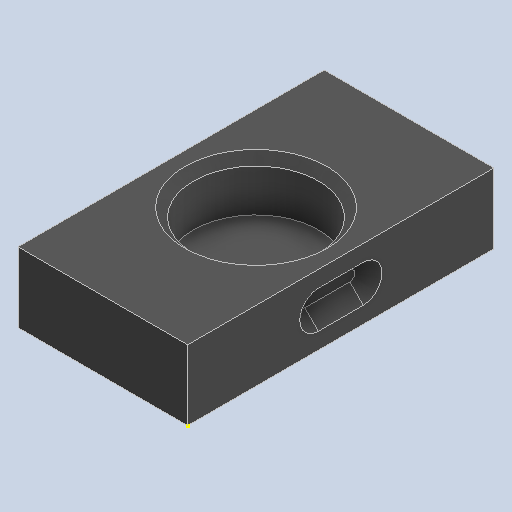
# Autodesk Inventor part: Pieza1
Saved by Autodesk Inventor 2026 (Build 300175050, 175E)
## iProperties
Created: 2025-09-26
Part Number: Pieza1
Material: Plastico PETG
Document SubType Name: Modeling
Designer: bello
Density: 1.27 g/cm^3
Appearance: Genérico
Author: bello
Autodesk Inventor part; units mm, degrees
ref_plane "YZ Plane" through (0, 0, 0) normal (1, 0, 0) x (0, 1, 0)
ref_plane "XZ Plane" through (0, 0, 0) normal (0, 1, 0) x (-1, 0, 0)
sketch "Boceto1" plane through (0, 0, 0) normal (0, 1, 0) x (-1, 0, 0)
  line L0 (0, 0) -> (-50.2, 0)
  line L1 (-50.2, 0) -> (-50.2, -90.6)
  line L2 (-50.2, -90.6) -> (0, -90.6)
  line L3 (0, -90.6) -> (0, 0)
  dimension "d0" = 50.2
  dimension "d1" = 90.6
  constraints: 8 end point, 2 parallel, 1 horizontal, 1 perpendicular
  measures "d0" distance of L2.end L1.end
  measures "d1" distance of L0.end L1.end
extrude "Extrusión1" add sketch "Boceto1" along normal blind 20.7
sketch "Boceto2" plane through (0, 20.7, 0) normal (0, 1, 0) x (1, 0, 0)
  line L0 (-14.4985, 45.3) -> (58.2485, 45.3)
  circle A0 centre (25.1, 45.3) radius 18.5
  line L1 (50.2, 90.6) -> (0, 90.6) projected
  point P0 (0, 0)
  dimension "d7" = 37
  dimension "d51" = 90.6
  dimension "d52" = 0
  constraints: 2 end point, 1 centre point
  measures "d7" diameter of A0
  measures "d51" diameter of L1 L0
  measures "d52" distance from line of A0.centre L0
extrude "Extrusión2" cut sketch "Boceto2" against normal blind 15
sketch "Boceto3" plane through (50.2, 0, 0) normal (1, 0, 0) x (0, 0, -1)
  line L0 (45.3, 28.8672) -> (45.3, -9.3744)
  line L1 (-5.2256, 10.35) -> (70.0589, 10.35)
  line L2 (38.65, 10.35) -> (51.95, 10.35) construction
  line L3 (38.65, 8.85) -> (51.95, 8.85)
  line L4 (51.95, 11.85) -> (38.65, 11.85)
  arc A0 (38.65, 11.85) -> (38.65, 8.85) centre (38.65, 10.35) ccw
  arc A1 (51.95, 8.85) -> (51.95, 11.85) centre (51.95, 10.35) ccw
  line L5 (90.6, 0) -> (90.6, 20.7) projected
  point P0 (0, 0)
  point P1 (45.3, 10.35)
  point P2 (53.45, 10.35)
  point P3 (37.15, 10.35)
  dimension "d11" = 16.3
  dimension "d12" = 3
  dimension "d13" = 0
  dimension "d53" = 45.3
  constraints: 12 end point, 6 point on circle, 4 tangent, 2 centre point, 2 point on line, 1 midpoint, 1 parallel
  measures "d11" distance of point (53.45, 10.35) point (37.15, 10.35)
  measures "d12" distance between parallel lines of L3 L4
  measures "d13" distance from line of point (45.3, 10.35) L0
  measures "d53" distance between parallel lines of L0 L5
extrude "Extrusión3" cut sketch "Boceto3" against normal blind 4
chamfer "Chaflán1" distance 4 angle 45 4 edges at (50.2, 8.85, -45.3) (50.2, 10.35, -37.15) (50.2, 11.85, -45.3) (50.2, 10.35, -53.45)
sketch "Boceto4" plane through (50.2, 0, 0) normal (1, 0, 0) x (0, 0, -1)
  point P0 (0, 0)
ref_plane "Plano de trabajo1" through (25.1, 0, 0) normal (1, 0, 0) x (0, 0, -1)
mirror "Simetría1" about plane through (25.1, 0, 0) normal (1, 0, 0) of "Extrusión3"
chamfer "Chaflán2" distance 4 angle 45 4 edges at (0, 11.85, -45.3) (0, 10.35, -37.15) (0, 8.85, -45.3) (0, 10.35, -53.45)
chamfer "Chaflán3" distance 2.5 angle 45 1 edges at (6.6, 20.7, -45.3)
sketch "Boceto5" plane through (0, 0, 0) normal (0, -1, 0) x (1, 0, 0)
  line L0 (25.1, 22.2035) -> (25.1, -86.3829)
  line L1 (-10.0483, -45.3) -> (59.9656, -45.3)
  circle A0 centre (6.05, -7.2) radius 3.2
  circle A1 centre (44.15, -7.2) radius 3.2
  circle A2 centre (44.15, -83.4) radius 3.2
  line L2 (0, 0) -> (50.2, 0) projected
  circle A3 centre (6.05, -83.4) radius 3.2
  dimension "d35" = 38.1
  dimension "d36" = 38.1
  dimension "d42" = 6.4
  dimension "d46" = 76.2
  dimension "d47" = 76.2
  dimension "d54" = 45.3
  constraints: 4 centre point, 4 end point, 3 equal radius, 2 vertical
  measures "d35" distance of A0.centre A1.centre
  measures "d36" diameter of A0.centre L0
  measures "d42" diameter of A0
  measures "d46" distance of A2.centre A1.centre
  measures "d47" diameter of A1.centre L1
  measures "d54" distance between parallel lines of L1 L2
extrude "Extrusión4" add sketch "Boceto5" along normal blind 4.2
fillet "Empalme1" radius 3.2 4 edges at (40.95, -4.2, -7.2) (2.85, -4.2, -7.2) (40.95, -4.2, -83.4) (2.85, -4.2, -83.4)
